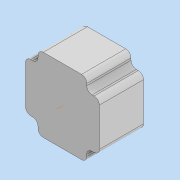
# Autodesk Inventor part: SERVO  KH56KM2U121 B
Saved by Autodesk Inventor 2021 (Build 250183000, 183)
## iProperties
Created: 2021-10-05
Part Number: SERVO  KH56KM2U121 B
Material: Generic
Document SubType Name: Modeling
Designer: 41601100
Density: 1 g/cm^3
Appearance: Default
Author: 41601100
Autodesk Inventor part; units mm, degrees
ref_plane "YZ Plane" through (0, 0, 0) normal (1, 0, 0) x (0, 1, 0)
ref_plane "XZ Plane" through (0, 0, 0) normal (0, 1, 0) x (-1, 0, 0)
ref_plane "XY Plane" through (0, 0, 0) normal (0, 0, 1) x (1, 0, 0)
sketch "Sketch1" plane through (0, 0, 0) normal (0, 0, 1) x (1, 0, 0)
  arc A0 (-24, 18.5) -> (-28, 14.5) centre (-24, 14.5) ccw
  line L0 (-28, 14.5) -> (-28, -14.5)
  arc A1 (-28, -14.5) -> (-24, -18.5) centre (-24, -14.5) ccw
  line L1 (-24, -18.5) -> (-22.5, -18.5)
  arc A2 (-18.5, -22.5) -> (-22.5, -18.5) centre (-22.5, -22.5) ccw
  line L2 (-18.5, -22.5) -> (-18.5, -24)
  arc A3 (-18.5, -24) -> (-14.5, -28) centre (-14.5, -24) ccw
  line L3 (-14.5, -28) -> (14.5, -28)
  arc A4 (14.5, -28) -> (18.5, -24) centre (14.5, -24) ccw
  line L4 (18.5, -24) -> (18.5, -22.5)
  arc A5 (22.5, -18.5) -> (18.5, -22.5) centre (22.5, -22.5) ccw
  line L5 (22.5, -18.5) -> (24, -18.5)
  arc A6 (24, -18.5) -> (28, -14.5) centre (24, -14.5) ccw
  line L6 (28, -14.5) -> (28, 14.5)
  arc A7 (28, 14.5) -> (24, 18.5) centre (24, 14.5) ccw
  line L7 (24, 18.5) -> (22.5, 18.5)
  arc A8 (18.5, 22.5) -> (22.5, 18.5) centre (22.5, 22.5) ccw
  line L8 (18.5, 22.5) -> (18.5, 24)
  arc A9 (18.5, 24) -> (14.5, 28) centre (14.5, 24) ccw
  line L9 (14.5, 28) -> (-14.5, 28)
  arc A10 (-14.5, 28) -> (-18.5, 24) centre (-14.5, 24) ccw
  line L10 (-18.5, 24) -> (-18.5, 22.5)
  arc A11 (-22.5, 18.5) -> (-18.5, 22.5) centre (-22.5, 22.5) ccw
  line L11 (-22.5, 18.5) -> (-24, 18.5)
  point P0 (0, 0)
  point P1 (0, 0)
  constraints: 24 end point, 24 point on circle, 12 centre point
extrude "Extrusion1" add sketch "Sketch1" along normal blind 33.5
body "Solid1"
